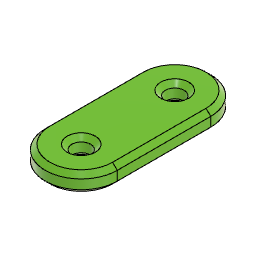
LoadingModuleClamp_M2 (Autodesk Fusion 360 design; units mm, degrees)
Autodesk Fusion 360 part; units mm, degrees
sketch "Skizze1" plane through (0, 0, 0) normal (0, 0, 1) x (1, 0, 0)
  line L0 (3.85, 0) -> (3.85, -10)
  line L1 (-3.85, -10) -> (-3.85, 0)
  arc A0 (-3.85, -10) -> (3.85, -10) centre (0, -10) ccw
  arc A1 (3.85, 0) -> (-3.85, 0) centre (0, 0) ccw
  circle A2 centre (0, 0) radius 1
  circle A3 centre (0, -10) radius 1
  dimension "d609" = 7.7
  dimension "d610" = 10
  dimension "d613" = 2
  constraint coincident A1.centre A2.centre
  constraint vertical L0
  constraint vertical L1
  constraint tangent L1 A1
  constraint tangent L0 A1
  constraint tangent L0 A0
  constraint tangent L1 A0
  constraint concentric A1 A2
  constraint concentric A0 A3
  constraint equal A2 A3
  measures "d609" diameter of A1
  measures "d610" distance of A1.centre A0.centre
  measures "d613" diameter of A2
extrude "Extrusion1" add sketch "Skizze1" along normal blind 2
chamfer "Fase1" distance 0.5 angle 45 12 edges at (0, -13.85, 0) (3.85, -5, 0) (0, 3.85, 0) (-3.85, -5, 0) (-0.9323, -9.6384, 0) (-0.9323, 0.3616, 0) (-0.9323, 0.3616, 2) (-0.9323, -9.6384, 2) (0, -13.85, 2) (3.85, -5, 2) (0, 3.85, 2) (-3.85, -5, 2)
equation "d609 = 8 mm - 0.3 mm"
named bodies: "LoadingModuleClamp"
